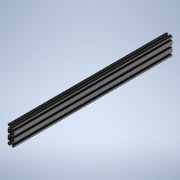
# Autodesk Inventor part: 25in 3x1 T Slot
Saved by Autodesk Inventor 2020 (Build 240168000, 168)
## iProperties
Created: 2020-01-07
Part Number: 25in 3x1 T Slot
Material: Steel, Alloy
Document SubType Name: Modeling
Designer: 393735
Density: 7.73 g/cm^3
Appearance: Semi-Polished
Author: 393735
Autodesk Inventor part; units mm, degrees
ref_plane "YZ Plane" through (0, 0, 0) normal (1, 0, 0) x (0, 1, 0)
ref_plane "XZ Plane" through (0, 0, 0) normal (0, 1, 0) x (-1, 0, 0)
ref_plane "XY Plane" through (0, 0, 0) normal (0, 0, 1) x (1, 0, 0)
sketch "Sketch1" plane through (0, 0, 0) normal (0, 0, 1) x (1, 0, 0)
  arc A0 (2.1336, 27.5336) -> (3.1496, 27.5336) centre (2.6416, 27.5336) ccw
  arc A1 (2.1336, 27.5336) -> (0, 25.4) centre (2.108, 25.4256) ccw
  arc A2 (0, 24.384) -> (0, 25.4) centre (0, 24.892) ccw
  line L0 (0, 24.384) -> (0, 21.1582)
  arc A3 (0, 20.1422) -> (0, 21.1582) centre (0, 20.6502) ccw
  line L1 (0, 20.1422) -> (0, 19.1359)
  arc A4 (0, 19.1359) -> (2.2098, 19.1359) centre (1.1049, 19.1359) ccw
  line L2 (2.2098, 19.1359) -> (2.2098, 21.3084)
  arc A5 (3.9442, 22.0268) -> (2.2098, 21.3084) centre (3.2258, 21.3084) ccw
  line L3 (3.9442, 22.0268) -> (7.2616, 18.7095)
  arc A6 (8.1915, 16.4644) -> (7.2616, 18.7095) centre (5.0165, 16.4644) ccw
  line L4 (8.1915, 16.4644) -> (8.1915, 13.2028)
  arc A7 (7.2616, 10.9577) -> (8.1915, 13.2028) centre (5.0165, 13.2028) ccw
  line L5 (7.2616, 10.9577) -> (3.9442, 7.6404)
  arc A8 (2.2098, 8.3588) -> (3.9442, 7.6404) centre (3.2258, 8.3588) ccw
  line L6 (2.2098, 8.3588) -> (2.2098, 10.5313)
  arc A9 (2.2098, 10.5313) -> (0, 10.5313) centre (1.1049, 10.5313) ccw
  line L7 (0, 10.5313) -> (0, 9.525)
  arc A10 (0, 8.509) -> (0, 9.525) centre (0, 9.017) ccw
  line L8 (0, 8.509) -> (0, 5.2832)
  arc A11 (0, 4.2672) -> (0, 5.2832) centre (0, 4.7752) ccw
  line L9 (0, 4.2672) -> (0, 0)
  arc A12 (0, -1.016) -> (0, 0) centre (0, -0.508) ccw
  line L10 (0, -1.016) -> (0, -4.2418)
  arc A13 (0, -5.2578) -> (0, -4.2418) centre (0, -4.7498) ccw
  line L11 (0, -5.2578) -> (0, -6.2641)
  arc A14 (0, -6.2641) -> (2.2098, -6.2641) centre (1.1049, -6.2641) ccw
  line L12 (2.2098, -6.2641) -> (2.2098, -4.0916)
  arc A15 (3.9442, -3.3732) -> (2.2098, -4.0916) centre (3.2258, -4.0916) ccw
  line L13 (3.9442, -3.3732) -> (7.2616, -6.6905)
  arc A16 (8.1915, -8.9356) -> (7.2616, -6.6905) centre (5.0165, -8.9356) ccw
  line L14 (8.1915, -8.9356) -> (8.1915, -12.1972)
  arc A17 (7.2616, -14.4423) -> (8.1915, -12.1972) centre (5.0165, -12.1972) ccw
  line L15 (7.2616, -14.4423) -> (3.9442, -17.7596)
  arc A18 (2.2098, -17.0412) -> (3.9442, -17.7596) centre (3.2258, -17.0412) ccw
  line L16 (2.2098, -17.0412) -> (2.2098, -14.8687)
  arc A19 (2.2098, -14.8687) -> (0, -14.8687) centre (1.1049, -14.8687) ccw
  line L17 (0, -14.8687) -> (0, -15.875)
  arc A20 (0, -16.891) -> (0, -15.875) centre (0, -16.383) ccw
  line L18 (0, -16.891) -> (0, -20.1168)
  arc A21 (0, -21.1328) -> (0, -20.1168) centre (0, -20.6248) ccw
  line L19 (0, -21.1328) -> (0, -25.4)
  arc A22 (0, -26.416) -> (0, -25.4) centre (0, -25.908) ccw
  line L20 (0, -26.416) -> (0, -29.6418)
  arc A23 (0, -30.6578) -> (0, -29.6418) centre (0, -30.1498) ccw
  line L21 (0, -30.6578) -> (0, -31.6641)
  arc A24 (0, -31.6641) -> (2.2098, -31.6641) centre (1.1049, -31.6641) ccw
  line L22 (2.2098, -31.6641) -> (2.2098, -29.4916)
  arc A25 (3.9442, -28.7732) -> (2.2098, -29.4916) centre (3.2258, -29.4916) ccw
  line L23 (3.9442, -28.7732) -> (7.2616, -32.0905)
  arc A26 (8.1915, -34.3356) -> (7.2616, -32.0905) centre (5.0165, -34.3356) ccw
  line L24 (8.1915, -34.3356) -> (8.1915, -37.5972)
  arc A27 (7.2616, -39.8423) -> (8.1915, -37.5972) centre (5.0165, -37.5972) ccw
  line L25 (7.2616, -39.8423) -> (3.9442, -43.1596)
  arc A28 (2.2098, -42.4412) -> (3.9442, -43.1596) centre (3.2258, -42.4412) ccw
  line L26 (2.2098, -42.4412) -> (2.2098, -40.2687)
  arc A29 (2.2098, -40.2687) -> (0, -40.2687) centre (1.1049, -40.2687) ccw
  line L27 (0, -40.2687) -> (0, -41.275)
  arc A30 (0, -42.291) -> (0, -41.275) centre (0, -41.783) ccw
  line L28 (0, -42.291) -> (0, -45.5168)
  arc A31 (0, -46.5328) -> (0, -45.5168) centre (0, -46.0248) ccw
  arc A32 (0, -46.5328) -> (2.1336, -48.6664) centre (2.108, -46.5584) ccw
  arc A33 (3.1496, -48.6664) -> (2.1336, -48.6664) centre (2.6416, -48.6664) ccw
  line L29 (3.1496, -48.6664) -> (6.3754, -48.6664)
  arc A34 (7.3914, -48.6664) -> (6.3754, -48.6664) centre (6.8834, -48.6664) ccw
  line L30 (7.3914, -48.6664) -> (8.3977, -48.6664)
  arc A35 (8.3977, -48.6664) -> (8.3977, -46.4566) centre (8.3977, -47.5615) ccw
  line L31 (8.3977, -46.4566) -> (6.2252, -46.4566)
  arc A36 (5.5068, -44.7222) -> (6.2252, -46.4566) centre (6.2252, -45.4406) ccw
  line L32 (5.5068, -44.7222) -> (8.8241, -41.4048)
  arc A37 (11.0692, -40.4749) -> (8.8241, -41.4048) centre (11.0692, -43.6499) ccw
  line L33 (11.0692, -40.4749) -> (14.3308, -40.4749)
  arc A38 (16.5759, -41.4048) -> (14.3308, -40.4749) centre (14.3308, -43.6499) ccw
  line L34 (16.5759, -41.4048) -> (19.8932, -44.7222)
  arc A39 (19.1748, -46.4566) -> (19.8932, -44.7222) centre (19.1748, -45.4406) ccw
  line L35 (19.1748, -46.4566) -> (17.0023, -46.4566)
  arc A40 (17.0023, -46.4566) -> (17.0023, -48.6664) centre (17.0023, -47.5615) ccw
  line L36 (17.0023, -48.6664) -> (18.0086, -48.6664)
  arc A41 (19.0246, -48.6664) -> (18.0086, -48.6664) centre (18.5166, -48.6664) ccw
  line L37 (19.0246, -48.6664) -> (22.2504, -48.6664)
  arc A42 (23.2664, -48.6664) -> (22.2504, -48.6664) centre (22.7584, -48.6664) ccw
  arc A43 (23.2664, -48.6664) -> (25.4, -46.5328) centre (23.292, -46.5584) ccw
  arc A44 (25.4, -45.5168) -> (25.4, -46.5328) centre (25.4, -46.0248) ccw
  line L38 (25.4, -45.5168) -> (25.4, -42.291)
  arc A45 (25.4, -41.275) -> (25.4, -42.291) centre (25.4, -41.783) ccw
  line L39 (25.4, -41.275) -> (25.4, -40.2687)
  arc A46 (25.4, -40.2687) -> (23.1902, -40.2687) centre (24.2951, -40.2687) ccw
  line L40 (23.1902, -40.2687) -> (23.1902, -42.4412)
  arc A47 (21.4558, -43.1596) -> (23.1902, -42.4412) centre (22.1742, -42.4412) ccw
  line L41 (21.4558, -43.1596) -> (18.1384, -39.8423)
  arc A48 (17.2085, -37.5972) -> (18.1384, -39.8423) centre (20.3835, -37.5972) ccw
  line L42 (17.2085, -37.5972) -> (17.2085, -34.3356)
  arc A49 (18.1384, -32.0905) -> (17.2085, -34.3356) centre (20.3835, -34.3356) ccw
  line L43 (18.1384, -32.0905) -> (21.4558, -28.7732)
  arc A50 (23.1902, -29.4916) -> (21.4558, -28.7732) centre (22.1742, -29.4916) ccw
  line L44 (23.1902, -29.4916) -> (23.1902, -31.6641)
  arc A51 (23.1902, -31.6641) -> (25.4, -31.6641) centre (24.2951, -31.6641) ccw
  line L45 (25.4, -31.6641) -> (25.4, -30.6578)
  arc A52 (25.4, -29.6418) -> (25.4, -30.6578) centre (25.4, -30.1498) ccw
  line L46 (25.4, -29.6418) -> (25.4, -26.416)
  arc A53 (25.4, -25.4) -> (25.4, -26.416) centre (25.4, -25.908) ccw
  line L47 (25.4, -25.4) -> (25.4, -21.1328)
  arc A54 (25.4, -20.1168) -> (25.4, -21.1328) centre (25.4, -20.6248) ccw
  line L48 (25.4, -20.1168) -> (25.4, -16.891)
  arc A55 (25.4, -15.875) -> (25.4, -16.891) centre (25.4, -16.383) ccw
  line L49 (25.4, -15.875) -> (25.4, -14.8687)
  arc A56 (25.4, -14.8687) -> (23.1902, -14.8687) centre (24.2951, -14.8687) ccw
  line L50 (23.1902, -14.8687) -> (23.1902, -17.0412)
  arc A57 (21.4558, -17.7596) -> (23.1902, -17.0412) centre (22.1742, -17.0412) ccw
  line L51 (21.4558, -17.7596) -> (18.1384, -14.4423)
  arc A58 (17.2085, -12.1972) -> (18.1384, -14.4423) centre (20.3835, -12.1972) ccw
  line L52 (17.2085, -12.1972) -> (17.2085, -8.9356)
  arc A59 (18.1384, -6.6905) -> (17.2085, -8.9356) centre (20.3835, -8.9356) ccw
  line L53 (18.1384, -6.6905) -> (21.4558, -3.3732)
  arc A60 (23.1902, -4.0916) -> (21.4558, -3.3732) centre (22.1742, -4.0916) ccw
  line L54 (23.1902, -4.0916) -> (23.1902, -6.2641)
  arc A61 (23.1902, -6.2641) -> (25.4, -6.2641) centre (24.2951, -6.2641) ccw
  line L55 (25.4, -6.2641) -> (25.4, -5.2578)
  arc A62 (25.4, -4.2418) -> (25.4, -5.2578) centre (25.4, -4.7498) ccw
  line L56 (25.4, -4.2418) -> (25.4, -1.016)
  arc A63 (25.4, 0) -> (25.4, -1.016) centre (25.4, -0.508) ccw
  line L57 (25.4, 0) -> (25.4, 4.2672)
  arc A64 (25.4, 5.2832) -> (25.4, 4.2672) centre (25.4, 4.7752) ccw
  line L58 (25.4, 5.2832) -> (25.4, 8.509)
  arc A65 (25.4, 9.525) -> (25.4, 8.509) centre (25.4, 9.017) ccw
  line L59 (25.4, 9.525) -> (25.4, 10.5313)
  arc A66 (25.4, 10.5313) -> (23.1902, 10.5313) centre (24.2951, 10.5313) ccw
  line L60 (23.1902, 10.5313) -> (23.1902, 8.3588)
  arc A67 (21.4558, 7.6404) -> (23.1902, 8.3588) centre (22.1742, 8.3588) ccw
  line L61 (21.4558, 7.6404) -> (18.1384, 10.9577)
  arc A68 (17.2085, 13.2028) -> (18.1384, 10.9577) centre (20.3835, 13.2028) ccw
  line L62 (17.2085, 13.2028) -> (17.2085, 16.4644)
  arc A69 (18.1384, 18.7095) -> (17.2085, 16.4644) centre (20.3835, 16.4644) ccw
  line L63 (18.1384, 18.7095) -> (21.4558, 22.0268)
  arc A70 (23.1902, 21.3084) -> (21.4558, 22.0268) centre (22.1742, 21.3084) ccw
  line L64 (23.1902, 21.3084) -> (23.1902, 19.1359)
  arc A71 (23.1902, 19.1359) -> (25.4, 19.1359) centre (24.2951, 19.1359) ccw
  line L65 (25.4, 19.1359) -> (25.4, 20.1422)
  arc A72 (25.4, 21.1582) -> (25.4, 20.1422) centre (25.4, 20.6502) ccw
  line L66 (25.4, 21.1582) -> (25.4, 24.384)
  arc A73 (25.4, 25.4) -> (25.4, 24.384) centre (25.4, 24.892) ccw
  arc A74 (25.4, 25.4) -> (23.2664, 27.5336) centre (23.292, 25.4256) ccw
  arc A75 (22.2504, 27.5336) -> (23.2664, 27.5336) centre (22.7584, 27.5336) ccw
  line L67 (22.2504, 27.5336) -> (19.0246, 27.5336)
  arc A76 (18.0086, 27.5336) -> (19.0246, 27.5336) centre (18.5166, 27.5336) ccw
  line L68 (18.0086, 27.5336) -> (17.0023, 27.5336)
  arc A77 (17.0023, 27.5336) -> (17.0023, 25.3238) centre (17.0023, 26.4287) ccw
  line L69 (17.0023, 25.3238) -> (19.1748, 25.3238)
  arc A78 (19.8932, 23.5894) -> (19.1748, 25.3238) centre (19.1748, 24.3078) ccw
  line L70 (19.8932, 23.5894) -> (16.5759, 20.272)
  arc A79 (14.3308, 19.3421) -> (16.5759, 20.272) centre (14.3308, 22.5171) ccw
  line L71 (14.3308, 19.3421) -> (11.0692, 19.3421)
  arc A80 (8.8241, 20.272) -> (11.0692, 19.3421) centre (11.0692, 22.5171) ccw
  line L72 (8.8241, 20.272) -> (5.5068, 23.5894)
  arc A81 (6.2252, 25.3238) -> (5.5068, 23.5894) centre (6.2252, 24.3078) ccw
  line L73 (6.2252, 25.3238) -> (8.3977, 25.3238)
  arc A82 (8.3977, 25.3238) -> (8.3977, 27.5336) centre (8.3977, 26.4287) ccw
  line L74 (8.3977, 27.5336) -> (7.3914, 27.5336)
  arc A83 (6.3754, 27.5336) -> (7.3914, 27.5336) centre (6.8834, 27.5336) ccw
  line L75 (6.3754, 27.5336) -> (3.1496, 27.5336)
  line L76 (3.2298, -24.9337) -> (8.8241, -30.528)
  arc A84 (2.7686, -23.8201) -> (3.2298, -24.9337) centre (4.3434, -23.8201) ccw
  line L77 (2.7686, -22.7127) -> (2.7686, -23.8201)
  arc A85 (3.2298, -21.5991) -> (2.7686, -22.7127) centre (4.3434, -22.7127) ccw
  line L78 (8.8241, -16.0048) -> (3.2298, -21.5991)
  arc A86 (11.0692, -15.0749) -> (8.8241, -16.0048) centre (11.0692, -18.2499) ccw
  line L79 (14.3308, -15.0749) -> (11.0692, -15.0749)
  arc A87 (16.5759, -16.0048) -> (14.3308, -15.0749) centre (14.3308, -18.2499) ccw
  line L80 (22.1702, -21.5991) -> (16.5759, -16.0048)
  arc A88 (22.6314, -22.7127) -> (22.1702, -21.5991) centre (21.0566, -22.7127) ccw
  line L81 (22.6314, -23.8201) -> (22.6314, -22.7127)
  arc A89 (22.1702, -24.9337) -> (22.6314, -23.8201) centre (21.0566, -23.8201) ccw
  line L82 (16.5759, -30.528) -> (22.1702, -24.9337)
  arc A90 (14.3308, -31.4579) -> (16.5759, -30.528) centre (14.3308, -28.2829) ccw
  line L83 (11.0692, -31.4579) -> (14.3308, -31.4579)
  arc A91 (8.8241, -30.528) -> (11.0692, -31.4579) centre (11.0692, -28.2829) ccw
  line L84 (3.2298, 0.4663) -> (8.8241, -5.128)
  arc A92 (2.7686, 1.5799) -> (3.2298, 0.4663) centre (4.3434, 1.5799) ccw
  line L85 (2.7686, 2.6873) -> (2.7686, 1.5799)
  arc A93 (3.2298, 3.8009) -> (2.7686, 2.6873) centre (4.3434, 2.6873) ccw
  line L86 (8.8241, 9.3952) -> (3.2298, 3.8009)
  arc A94 (11.0692, 10.3251) -> (8.8241, 9.3952) centre (11.0692, 7.1501) ccw
  line L87 (14.3308, 10.3251) -> (11.0692, 10.3251)
  arc A95 (16.5759, 9.3952) -> (14.3308, 10.3251) centre (14.3308, 7.1501) ccw
  line L88 (22.1702, 3.8009) -> (16.5759, 9.3952)
  arc A96 (22.6314, 2.6873) -> (22.1702, 3.8009) centre (21.0566, 2.6873) ccw
  line L89 (22.6314, 1.5799) -> (22.6314, 2.6873)
  arc A97 (22.1702, 0.4663) -> (22.6314, 1.5799) centre (21.0566, 1.5799) ccw
  line L90 (16.5759, -5.128) -> (22.1702, 0.4663)
  arc A98 (14.3308, -6.0579) -> (16.5759, -5.128) centre (14.3308, -2.8829) ccw
  line L91 (11.0692, -6.0579) -> (14.3308, -6.0579)
  arc A99 (8.8241, -5.128) -> (11.0692, -6.0579) centre (11.0692, -2.8829) ccw
  circle A100 centre (12.7, 14.8336) radius 2.6035
  circle A101 centre (12.7, -10.5664) radius 2.6035
  circle A102 centre (12.7, -35.9664) radius 2.6035
  constraints: 200 point on circle, 184 end point, 103 centre point
extrude "Extrusion1" add sketch "Sketch1" along normal blind 660.4
body "Solid1"
